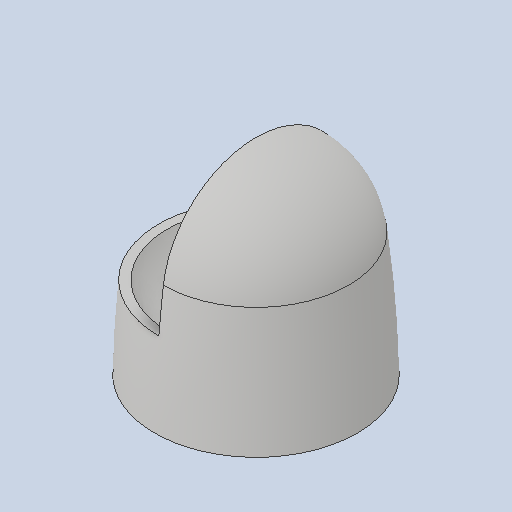
# Autodesk Inventor part: ч ASY human dummy 01
Saved by Autodesk Inventor 2024.2 (Build 282272000, 272)
## iProperties
Created: 2019-08-19
Part Number: ч ASY human dummy 01
Material: Типовые
Document SubType Name: Modeling
Designer: admin
Density: 1 g/cm^3
Appearance: По умолчанию
Author: admin
Autodesk Inventor part; units mm, degrees
ref_plane "YZ Plane" through (0, 0, 0) normal (1, 0, 0) x (0, 1, 0)
ref_plane "XZ Plane" through (0, 0, 0) normal (0, 1, 0) x (-1, 0, 0)
ref_plane "XY Plane" through (0, 0, 0) normal (0, 0, 1) x (1, 0, 0)
sketch "Эскиз1" plane through (0, 0, 0) normal (0, 0, 1) x (1, 0, 0)
  arc A0 (49.6078, 6.25) -> (0, 50) centre (0, 0) ccw
  line L0 (0, 0) -> (0, -250)
  circle A1 centre (0, -250) radius 25
  arc A2 (23.7255, -257.8804) -> (54.25, -60) centre (-545.6862, -68.75) ccw construction
  line L1 (54.25, -60) -> (0, -60)
  arc A3 (0, -50) -> (49.6078, 6.25) centre (0, 0) ccw construction
  line L2 (0, 0) -> (0, 50)
  arc A4 (0, 50) -> (0, -50) centre (0, 0) ccw construction
  arc A5 (54.25, -60) -> (49.6078, 6.25) centre (-545.6862, -68.75) ccw
  dimension "d2" = 50
  dimension "d0" = 100
  dimension "d1" = 250
  dimension "d3" = 600
  dimension "d4" = 60
  constraints: 10 point on circle, 6 end point, 5 centre point, 2 coincident, 2 point on line, 2 vertical, 1 perpendicular, 1 tangent, 4 other
  measures "d0" diameter of A0
  measures "d1" distance of L0.start L0.end
  measures "d3" radius of A2
  measures "d4" distance from line of L1 point (0, 0)
revolve "Вращение1" add sketch "Эскиз1" angle 360 about axis through (0, 0, 0) along (0, -1, 0) contours A5 L1 L0 L2 A0
sketch "Эскиз2" plane through (0, 0, 0) normal (1, 0, 0) x (0, 1, 0)
  line L0 (6.25, 49.6078) -> (6.25, -49.6078) construction
  arc A0 (0, -50) -> (0, 50) centre (0, 0) ccw construction
  line L1 (0, -50) -> (0, 50)
  arc A1 (0, 50) -> (0, -50) centre (0, 0) ccw
  dimension "d6" = 100
  constraints: 4 point on circle, 2 centre point, 2 coincident, 2 end point, 1 midpoint, 1 vertical
  measures "d6" diameter of A0
revolve "Вращение2" cut sketch "Эскиз2" angle 180 about axis through (0, 0, -50) along (0, 0, -1)
sketch "Эскиз3" plane through (0, 0, 0) normal (0, 0, 1) x (1, 0, 0)
  line L0 (0, 6.25) -> (0, 50) projected
  arc A0 (-49.6078, 6.25) -> (-54.25, -60) centre (545.6862, -68.75) ccw projected
  line L1 (0, 50) -> (-52, 50)
  line L2 (-52, 50) -> (-52, -16.1078)
  line L3 (-52, -16.1078) -> (0, -16.1078)
  line L4 (0, -16.1078) -> (0, 50)
  point P0 (0, 0)
  dimension "d11" = 52
  constraints: 8 end point, 2 parallel, 1 horizontal, 1 perpendicular, 1 point on circle
  measures "d11" distance of L0.end L1.end
extrude "Выдавливание1" cut sketch "Эскиз3" along normal through all both and the other way through all
